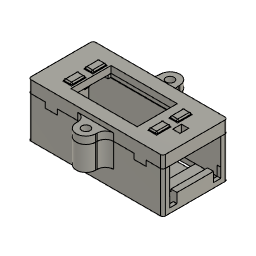
PicoCase - Display - Mounts - IO (Autodesk Fusion 360 design; units mm, degrees)
part number: PicoCase - Display - ExtraIO - Mounting Brackets - Buttons
Autodesk Fusion 360 part; units mm, degrees
note: some values were not read from the file. Set by a fixed rule: which sketch regions a step uses.
sketch "Base" plane through (0, 0, 0) normal (0, 0, 1) x (1, 0, 0)
  line L0 (1, 0) -> (54.5, 0)
  line L1 (55.5, 1) -> (55.5, 25.7)
  line L2 (54.5, 26.7) -> (1, 26.7)
  line L3 (0, 25.7) -> (0, 1)
  arc A0 (1, 26.7) -> (0, 25.7) centre (1, 25.7) ccw
  arc A1 (55.5, 25.7) -> (54.5, 26.7) centre (54.5, 25.7) ccw
  arc A2 (54.5, 0) -> (55.5, 1) centre (54.5, 1) ccw
  arc A3 (0, 1) -> (1, 0) centre (1, 1) ccw
  line L4 (1, 25.7) -> (1, 1)
  line L5 (54, 23.9) -> (55.5, 23.9)
  line L6 (53, 2.8) -> (55.5, 2.8)
  line L7 (1, 25.7) -> (53, 25.7)
  line L8 (53, 25.7) -> (53, 23.9)
  line L9 (53, 23.9) -> (1, 23.9)
  line L10 (1, 23.9) -> (1, 25.7)
  line L11 (1, 23.9) -> (54, 23.9)
  line L12 (54, 23.89) -> (1, 23.89)
  line L13 (1, 23.89) -> (1, 23.9)
  line L14 (1, 23.89) -> (54, 23.89)
  line L15 (54, 23.89) -> (54, 20.89)
  line L16 (54, 20.89) -> (1, 20.89)
  line L17 (1, 20.89) -> (1, 23.89)
  line L18 (54, 23.9) -> (54, 23.89)
  line L19 (1, 20.89) -> (53, 20.89)
  line L20 (53, 20.89) -> (53, 5.81)
  line L21 (53, 5.81) -> (1, 5.81)
  line L22 (1, 5.81) -> (1, 20.89)
  line L23 (48, 20.89) -> (53, 20.89)
  line L24 (53, 20.89) -> (53, 5.81)
  line L25 (53, 5.81) -> (48, 5.81)
  line L26 (48, 5.81) -> (48, 20.89)
  line L27 (1, 2.8) -> (53, 2.8)
  line L28 (53, 2.8) -> (53, 1)
  line L29 (53, 1) -> (1, 1)
  line L30 (1, 1) -> (1, 2.8)
  line L31 (1, 2.81) -> (54, 2.81)
  line L32 (54, 2.81) -> (54, 2.8)
  line L33 (54, 2.8) -> (1, 2.8)
  line L34 (1, 2.8) -> (1, 2.81)
  line L35 (1, 5.81) -> (54, 5.81)
  line L36 (54, 5.81) -> (54, 2.81)
  line L37 (54, 2.81) -> (1, 2.81)
  line L38 (1, 2.81) -> (1, 5.81)
  circle A4 centre (27.75, 30.7) radius 1.7
  line L39 (31.75, 30.7) -> (31.75, 26.7)
  line L40 (23.75, 30.7) -> (23.75, 26.7)
  arc A5 (31.75, 30.7) -> (23.75, 30.7) centre (27.75, 30.7) ccw
  line L41 (27.75, 30.7) -> (27.75, 26.7) construction
  circle A6 centre (27.75, -4) radius 1.7
  line L42 (27.75, -4) -> (27.75, 0) construction
  line L43 (23.75, -4) -> (23.75, 0)
  line L44 (31.75, -4) -> (31.75, 0)
  arc A7 (23.75, -4) -> (31.75, -4) centre (27.75, -4) ccw
  line L45 (0, 0) -> (75, 0) construction
  line L46 (75, 0) -> (130.5, 0)
  line L47 (130.5, 0) -> (130.5, 26.7)
  line L48 (130.5, 26.7) -> (75, 26.7)
  line L49 (75, 26.7) -> (75, 0)
  line L50 (81.9375, 26.7) -> (86.9375, 26.7)
  line L51 (86.9375, 26.7) -> (86.9375, 25.7)
  line L52 (86.9375, 25.7) -> (81.9375, 25.7)
  line L53 (81.9375, 25.7) -> (81.9375, 26.7)
  line L54 (86.9375, 1) -> (86.9375, 0)
  line L55 (81.9375, 0) -> (81.9375, 1)
  line L56 (81.9375, 1) -> (86.9375, 1)
  line L57 (86.9375, 0) -> (81.9375, 0)
  line L58 (118.5625, 26.7) -> (123.5625, 26.7)
  line L59 (123.5625, 26.7) -> (123.5625, 25.7)
  line L60 (123.5625, 25.7) -> (118.5625, 25.7)
  line L61 (118.5625, 25.7) -> (118.5625, 26.7)
  line L62 (118.5625, 1) -> (123.5625, 1)
  line L63 (123.5625, 1) -> (123.5625, 0)
  line L64 (123.5625, 0) -> (118.5625, 0)
  line L65 (118.5625, 0) -> (118.5625, 1)
  line L66 (75, 23.3625) -> (76, 23.3625)
  line L67 (76, 23.3625) -> (76, 18.3625)
  line L68 (76, 18.3625) -> (75, 18.3625)
  line L69 (75, 18.3625) -> (75, 23.3625)
  line L70 (75, 8.3375) -> (76, 8.3375)
  line L71 (76, 8.3375) -> (76, 3.3375)
  line L72 (76, 3.3375) -> (75, 3.3375)
  line L73 (75, 3.3375) -> (75, 8.3375)
  line L74 (86.7, 22.35) -> (118.2, 22.35)
  line L75 (118.2, 22.35) -> (118.2, 4.35)
  line L76 (118.2, 4.35) -> (86.7, 4.35)
  line L77 (86.7, 4.35) -> (86.7, 22.35)
  line L78 (75, 13.35) -> (130.5, 13.35) construction
  line L79 (82.7, 21.2) -> (82.7, 5.7) construction
  line L80 (82.7, 21.2) -> (86.7, 21.2)
  line L81 (86.7, 21.2) -> (86.7, 14.4)
  line L82 (86.7, 14.4) -> (82.7, 14.4)
  line L83 (82.7, 14.4) -> (82.7, 21.2)
  line L84 (82.7, 12.5) -> (86.7, 12.5)
  line L85 (86.7, 12.5) -> (86.7, 5.7)
  line L86 (86.7, 5.7) -> (82.7, 5.7)
  line L87 (82.7, 5.7) -> (82.7, 12.5)
  line L88 (118.2, 21.2) -> (122.2, 21.2)
  line L89 (122.2, 21.2) -> (122.2, 14.4)
  line L90 (122.2, 14.4) -> (118.2, 14.4)
  line L91 (118.2, 14.4) -> (118.2, 21.2)
  line L92 (118.2, 12.5) -> (122.2, 12.5)
  line L93 (122.2, 12.5) -> (122.2, 5.7)
  line L94 (122.2, 5.7) -> (118.2, 5.7)
  line L95 (118.2, 5.7) -> (118.2, 12.5)
  line L96 (123, 15.15) -> (126, 15.15)
  line L97 (126, 15.15) -> (126, 11.55)
  line L98 (126, 11.55) -> (123, 11.55)
  line L99 (123, 11.55) -> (123, 15.15)
  line L100 (102.45, 22.35) -> (102.45, 4.35) construction
  line L101 (118.2, 20.8) -> (121.8, 20.8)
  line L102 (121.8, 20.8) -> (121.8, 14.8)
  line L103 (121.8, 14.8) -> (118.2, 14.8)
  line L104 (118.2, 12.1) -> (121.8, 12.1)
  line L105 (121.8, 12.1) -> (121.8, 6.1)
  line L106 (121.8, 6.1) -> (118.2, 6.1)
  line L107 (86.7, 20.8) -> (83.1, 20.8)
  line L108 (83.1, 20.8) -> (83.1, 14.8)
  line L109 (83.1, 14.8) -> (86.7, 14.8)
  line L110 (86.7, 12.1) -> (83.1, 12.1)
  line L111 (83.1, 12.1) -> (83.1, 6.1)
  line L112 (83.1, 6.1) -> (86.7, 6.1)
  line L113 (87.5, 21.6) -> (114.8, 21.6)
  line L114 (114.8, 21.6) -> (114.8, 5.1)
  line L115 (114.8, 5.1) -> (87.5, 5.1)
  line L116 (87.5, 5.1) -> (87.5, 21.6)
  line L117 (101.15, 21.6) -> (101.15, 5.1) construction
  circle A8 centre (102.75, -4) radius 1.7
  line L118 (102.75, -4) -> (102.75, 0) construction
  line L119 (98.75, -4) -> (98.75, 0)
  line L120 (106.75, -4) -> (106.75, 0)
  arc A9 (98.75, -4) -> (106.75, -4) centre (102.75, -4) ccw
  circle A10 centre (102.75, 30.7) radius 1.7
  line L121 (102.75, 30.7) -> (102.75, 26.7) construction
  line L122 (98.75, 30.7) -> (98.75, 26.7)
  line L123 (106.75, 30.7) -> (106.75, 26.7)
  arc A11 (106.75, 30.7) -> (98.75, 30.7) centre (102.75, 30.7) ccw
  line L124 (0, 0) -> (0, -20) construction
  line L125 (0, -20) -> (0.4, -20)
  line L126 (0.4, -20) -> (0.4, -23.4)
  line L127 (0.4, -23.4) -> (0, -23.4)
  line L128 (0, -23.4) -> (0, -20)
  line L129 (0, -23.4) -> (6.6, -23.4)
  line L130 (6.2, -23.4) -> (6.6, -23.4)
  line L131 (6.6, -23.4) -> (6.6, -20)
  line L132 (6.6, -20) -> (6.2, -20)
  line L133 (6.2, -20) -> (6.2, -23.4)
  line L134 (0.4, -20) -> (6.2, -20)
  line L135 (85.7, 14.4) -> (85.7, 12.5)
  point P0 (55.5, 0)
  point P1 (55.5, 26.7)
  point P2 (0, 26.7)
  point P3 (27.75, 26.7)
  point P4 (27.75, 0)
  point P5 (123, 13.35)
  point P6 (102.45, 13.35)
  point P7 (101.15, 13.35)
  dimension "d27" = 1
  dimension "d31" = 52
  dimension "d32" = 1.8
  dimension "d33" = 0.01
  dimension "d35" = 1
  dimension "d37" = 1
  dimension "d38" = 53
  dimension "d39" = 3
  dimension "d40" = 5
  dimension "d41" = 52
  dimension "d43" = 1
  dimension "d44" = 1.8
  dimension "d45" = 0.01
  dimension "d46" = 3
  dimension "d47" = 53
  dimension "d48" = 52
  dimension "d91" = 2.5
  dimension "d93" = 24.7
  dimension "d114" = 21.1
  dimension "d115" = 26.7
  dimension "d117" = 1.5
  dimension "d118" = 55.5
  dimension "d119" = 8
  dimension "d122" = 3.4
  dimension "d123" = 4
  dimension "d124" = 4
  dimension "d125" = 3.4
  dimension "d126" = 8
  dimension "d127" = 4
  dimension "d128" = 4
  dimension "d159" = 75
  dimension "d160" = 26.7
  dimension "d161" = 55.5
  dimension "d162" = 1
  dimension "d163" = 5
  dimension "d164" = 6.9375
  dimension "d165" = 1
  dimension "d166" = 5
  dimension "d167" = 6.9375
  dimension "d168" = 5
  dimension "d169" = 1
  dimension "d170" = 6.9375
  dimension "d171" = 6.9375
  dimension "d172" = 5
  dimension "d173" = 1
  dimension "d174" = 5
  dimension "d175" = 3.3375
  dimension "d176" = 1
  dimension "d177" = 5
  dimension "d178" = 3.3375
  dimension "d179" = 1
  dimension "d183" = 18
  dimension "d187" = 7.7
  dimension "d192" = 6.8
  dimension "d193" = 4
  dimension "d200" = 6.8
  dimension "d201" = 4
  dimension "d206" = 6.8
  dimension "d207" = 4
  dimension "d208" = 4
  dimension "d209" = 6.8
  dimension "d210" = 0
  dimension "d215" = 3
  dimension "d216" = 3.6
  dimension "d225" = 5.5
  dimension "d227" = 5.5
  dimension "d230" = 5.7
  dimension "d231" = 5.7
  dimension "d237" = 48
  dimension "d241" = 0.4
  dimension "d242" = 0.4
  dimension "d243" = 0.4
  dimension "d244" = 0.4
  dimension "d245" = 0.4
  dimension "d246" = 0.4
  dimension "d247" = 0.4
  dimension "d248" = 0.4
  dimension "d249" = 0.4
  dimension "d250" = 0.4
  dimension "d251" = 0.4
  dimension "d252" = 0.4
  dimension "d265" = 16.5
  dimension "d266" = 27.3
  dimension "d300" = 3.4
  dimension "d301" = 8
  dimension "d302" = 4
  dimension "d303" = 4
  dimension "d304" = 8
  dimension "d305" = 3.4
  dimension "d306" = 4
  dimension "d307" = 4
  dimension "d314" = 3.4
  dimension "d319" = 0.4
  dimension "d321" = 0.4
  dimension "d322" = 20
  dimension "d354" = 8.3
  dimension "d356" = 12.5
  dimension "d357" = 3
  dimension "d364" = 5.8
  constraint horizontal L0
  constraint vertical L1
  constraint horizontal L2
  constraint vertical L3
  constraint coincident P2 L2
  constraint coincident P2 L3
  constraint tangent L2 A0
  constraint tangent L3 A0
  constraint coincident P1 L1
  constraint coincident P1 L2
  constraint tangent L1 A1
  constraint tangent L2 A1
  constraint equal A0 A1
  constraint coincident P0 L0
  constraint coincident P0 L1
  constraint tangent L0 A2
  constraint tangent L1 A2
  constraint equal A0 A2
  constraint tangent L0 A3
  constraint tangent L3 A3
  constraint equal A0 A3
  constraint coincident L45.start L3
  constraint coincident L45.start L0
  constraint coincident L1 L5.end
  constraint perpendicular L1 L5
  constraint coincident L1 L6.end
  constraint perpendicular L1 L6
  constraint horizontal L7
  constraint vertical L8
  constraint horizontal L9
  constraint vertical L10
  constraint collinear L4 L10
  constraint horizontal L11
  constraint horizontal L12
  constraint vertical L13
  constraint collinear L4 L13
  constraint collinear L9 L11
  constraint horizontal L14
  constraint vertical L15
  constraint horizontal L16
  constraint vertical L17
  constraint collinear L4 L17
  constraint parallel L3 L4
  constraint coincident L5 L8.end
  constraint collinear L12 L14
  constraint perpendicular L12 L18
  constraint coincident L9 L5.start
  constraint coincident L12.start L14.end
  constraint horizontal L19
  constraint vertical L20
  constraint horizontal L21
  constraint vertical L22
  constraint collinear L4 L22
  constraint horizontal L23
  constraint vertical L24
  constraint horizontal L25
  constraint vertical L26
  constraint collinear L19 L23
  constraint collinear L20 L24
  constraint collinear L21 L25
  constraint collinear L16 L19
  constraint horizontal L27
  constraint vertical L28
  constraint horizontal L29
  constraint vertical L30
  constraint collinear L4 L30
  constraint coincident L6 L27.end
  constraint coincident L6.start L27.end
  constraint horizontal L31
  constraint vertical L32
  constraint horizontal L33
  constraint vertical L34
  constraint collinear L4 L34
  constraint collinear L27 L33
  constraint horizontal L35
  constraint vertical L36
  constraint horizontal L37
  constraint vertical L38
  constraint collinear L4 L38
  constraint coincident L32 L31.end
  constraint collinear L31 L37
  constraint collinear L21 L35
  constraint coincident A3.centre L29
  constraint concentric A4 A5
  constraint tangent L2 A5
  constraint coincident L2 L39.end
  constraint tangent L39 A5
  constraint coincident L2 L40.end
  constraint tangent L40 A5
  constraint coincident A4.centre A5.centre
  constraint coincident L2 P3
  constraint perpendicular L2 L41
  constraint midpoint L2 P3
  constraint coincident L41 P3
  constraint concentric A6 A7
  constraint coincident A6.centre L42.start
  constraint coincident L0 P4
  constraint perpendicular L0 L42
  constraint midpoint L0 P4
  constraint coincident L42 P4
  constraint tangent L0 A7
  constraint coincident L0 L43.end
  constraint tangent L43 A7
  constraint coincident L0 L44.end
  constraint tangent L44 A7
  constraint coincident L45.start L124.start
  constraint parallel L0 L45
  constraint horizontal L46
  constraint vertical L47
  constraint horizontal L48
  constraint vertical L49
  constraint horizontal L50
  constraint vertical L51
  constraint horizontal L52
  constraint vertical L53
  constraint collinear L48 L50
  constraint horizontal L56
  constraint vertical L54
  constraint horizontal L57
  constraint vertical L55
  constraint collinear L46 L57
  constraint horizontal L58
  constraint vertical L59
  constraint horizontal L60
  constraint vertical L61
  constraint horizontal L62
  constraint vertical L63
  constraint horizontal L64
  constraint vertical L65
  constraint collinear L48 L58
  constraint collinear L46 L64
  constraint horizontal L66
  constraint vertical L67
  constraint horizontal L68
  constraint vertical L69
  constraint horizontal L70
  constraint vertical L71
  constraint horizontal L72
  constraint vertical L73
  constraint collinear L49 L69
  constraint collinear L49 L73
  constraint horizontal L74
  constraint vertical L75
  constraint horizontal L76
  constraint vertical L77
  constraint midpoint L49 L78.start
  constraint midpoint L47 L78.end
  constraint perpendicular L78 L79
  constraint horizontal L80
  constraint vertical L81
  constraint horizontal L82
  constraint vertical L83
  constraint coincident L79.start L80
  constraint collinear L79 L83
  constraint horizontal L84
  constraint vertical L85
  constraint horizontal L86
  constraint vertical L87
  constraint coincident L79.end L86
  constraint collinear L79 L87
  constraint horizontal L88
  constraint vertical L89
  constraint horizontal L90
  constraint vertical L91
  constraint horizontal L92
  constraint vertical L93
  constraint horizontal L94
  constraint vertical L95
  constraint collinear L91 L95
  constraint horizontal L96
  constraint vertical L97
  constraint horizontal L98
  constraint vertical L99
  constraint midpoint L99 P5
  constraint coincident L78 P5
  constraint midpoint L74 L100.start
  constraint midpoint L76 L100.end
  constraint midpoint L100 P6
  constraint coincident L78 P6
  constraint horizontal L101
  constraint perpendicular L101 L102
  constraint perpendicular L102 L103
  constraint coincident L91 L101.start
  constraint coincident L91 L103.end
  constraint coincident L95 L104.start
  constraint perpendicular L95 L104
  constraint perpendicular L104 L105
  constraint coincident L95 L106.end
  constraint perpendicular L95 L106
  constraint coincident L81 L107.start
  constraint perpendicular L81 L107
  constraint perpendicular L107 L108
  constraint coincident L81 L109.end
  constraint perpendicular L81 L109
  constraint coincident L85 L110.start
  constraint perpendicular L85 L110
  constraint perpendicular L110 L111
  constraint coincident L85 L112.end
  constraint perpendicular L85 L112
  constraint collinear L77 L81
  constraint collinear L75 L91
  constraint horizontal L113
  constraint vertical L114
  constraint horizontal L115
  constraint vertical L116
  constraint midpoint L113 L117.start
  constraint midpoint L115 L117.end
  constraint midpoint L117 P7
  constraint coincident L78 P7
  constraint concentric A8 A9
  constraint coincident A8.centre L118.start
  constraint midpoint L46 L118.end
  constraint perpendicular L46 L118
  constraint coincident L46 L119.end
  constraint tangent L119 A9
  constraint coincident L46 L120.end
  constraint tangent L120 A9
  constraint perpendicular L46 L119
  constraint concentric A10 A11
  constraint coincident A10.centre L121.start
  constraint midpoint L48 L121.end
  constraint perpendicular L48 L121
  constraint coincident L48 L122.end
  constraint perpendicular L48 L122
  constraint coincident L48 L123.end
  constraint tangent L123 A11
  constraint perpendicular L48 L123
  constraint perpendicular L45 L124
  constraint horizontal L125
  constraint vertical L126
  constraint horizontal L127
  constraint vertical L128
  constraint horizontal L129
  constraint horizontal L130
  constraint vertical L131
  constraint horizontal L132
  constraint vertical L133
  constraint coincident L127.end L128.start
  constraint coincident L129.end L130.end
  constraint coincident L124.end L125.start
  constraint parallel L129 L134
  constraint coincident L82 L135.start
  constraint coincident L84 L135.end
  constraint perpendicular L84 L135
  measures "d27" radius of A0
  measures "d31" distance of L8 L10
  measures "d32" distance of L7 L9
  measures "d33" distance of L11 L12
  measures "d35" distance of L3 L4
  measures "d37" distance of L2 L7
  measures "d38" distance of L15.end L16.end
  measures "d39" distance of L14 L16
  measures "d40" distance of L24 L26
  measures "d41" distance of L28 L30
  measures "d43" distance of L0 L29
  measures "d44" distance of L27 L29
  measures "d45" distance of L31 L33
  measures "d46" distance of L35 L37
  measures "d47" distance of L36 L38
  measures "d48" distance of L22 L24
  measures "d91" distance of L1 L20
  measures "d93" distance of L7 L29
  measures "d114" distance of L9 L27
  measures "d115" distance of L0 L2
  measures "d117" distance of L1 L15
  measures "d118" distance of L1 L3
  measures "d119" diameter of A5
  measures "d122" diameter of A4
  measures "d123" vertical distance of L39.start L39.end
  measures "d124" vertical distance of L40.start L40.end
  measures "d125" diameter of A6
  measures "d126" diameter of A7
  measures "d127" vertical distance of L43.start L43.end
  measures "d128" vertical distance of L44.start L44.end
  measures "d159" distance of L45.start L45.end
  measures "d160" distance of L45.end L48.end
  measures "d161" distance of L47.end L48.end
  measures "d162" distance of L50.end L51.end
  measures "d163" distance of L51 L53
  measures "d164" distance of L49 L53
  measures "d165" distance of L54.end L54.start
  measures "d166" distance of L54 L55
  measures "d167" distance of L49 L55
  measures "d168" distance of L59 L61
  measures "d169" distance of L58 L60
  measures "d170" distance of L47 L59
  measures "d171" distance of L47 L63
  measures "d172" distance of L63 L65
  measures "d173" distance of L62 L64
  measures "d174" distance of L66 L68
  measures "d175" distance of L48 L66
  measures "d176" distance of L67 L69
  measures "d177" distance of L70 L72
  measures "d178" distance of L46 L72
  measures "d179" distance of L71 L73
  measures "d183" distance of L74 L76
  measures "d187" distance of L49 L79
  measures "d192" distance of L80 L82
  measures "d193" distance of L81 L83
  measures "d200" distance of L84 L86
  measures "d201" distance of L85 L87
  measures "d206" distance of L88 L90
  measures "d207" distance of L89 L91
  measures "d208" distance of L93 L95
  measures "d209" distance of L92 L94
  measures "d210" distance of L75 L91
  measures "d215" distance of L97 L99
  measures "d216" distance of L96 L98
  measures "d225" distance of L48 L88
  measures "d227" distance of L48 L80
  measures "d230" distance of L46 L94
  measures "d231" distance of L46 L86
  measures "d237" distance of L49 L99
  measures "d241" distance of L88 L101
  measures "d242" distance of L89 L102
  measures "d243" distance of L90 L103
  measures "d244" distance of L92 L104
  measures "d245" distance of L93 L105
  measures "d246" distance of L94 L106
  measures "d247" distance of L80 L107
  measures "d248" distance of L79 L108
  measures "d249" distance of L82 L109
  measures "d250" distance of L84 L110
  measures "d251" distance of L79 L111
  measures "d252" distance of L86 L112
  measures "d265" distance of L113 L115
  measures "d266" distance of L114 L116
  measures "d300" diameter of A8
  measures "d301" diameter of A9
  measures "d302" vertical distance of L119.start L119.end
  measures "d303" vertical distance of L120.start L120.end
  measures "d304" diameter of A11
  measures "d305" diameter of A10
  measures "d306" distance of L123.start L123.end
  measures "d307" distance of L122.start L122.end
  measures "d314" distance of L125.end L126.end
  measures "d319" distance of L126 L128
  measures "d321" distance of L131 L133
  measures "d322" distance of L45.start L124.end
  measures "d354" distance of L47 L89
  measures "d356" distance of L49 L116
  measures "d357" distance of L79 L135
  measures "d364" distance of L126 L133
extrude "Extrude1" add sketch "Base" along normal blind 17 contours L0 L1 L2 L3 A0 A1 A2 A3 L4 L5 L6 L7 L8 L10 L11 L13 L17 L22 L28 L29 L30 L33 L34 L38 makes body 1
extrude "Extrude2" add sketch "Base" along normal blind 15.25 contours L4 L7 L8 L9 L10 L11 bodies 1
extrude "Extrude3" add sketch "Base" along normal blind 2 contours L4 L9 L11 L12 L13 L14 L18 bodies 1
extrude "Extrude4" add sketch "Base" along normal blind 2 contours L4 L16 L19 L21 L22 L26 L35 bodies 1
extrude "Extrude5" add sketch "Base" along normal blind 5 contours L16 L19 L20 L21 L23 L24 L25 L26 L35 bodies 1
extrude "Extrude6" add sketch "Base" along normal blind 2 contours L4 L6 L27 L31 L32 L33 L34 L37 bodies 1
extrude "Extrude7" add sketch "Base" along normal blind 15.25 contours L4 L27 L28 L29 L30 L33 bodies 1
extrude "Extrude8" add sketch "Base" along normal blind 6 contours L1 L5 L6 L15 L16 L18 L20 L24 L32 L35 L36 bodies 1
sketch "Insert End" plane through (55.5, 0, 0) normal (1, 0, 0) x (0, 1, 0)
  line L0 (1, 0) -> (25.7, 0)
  line L1 (25.7, 0) -> (25.7, 17)
  line L2 (25.7, 17) -> (23.9, 17)
  line L3 (23.9, 17) -> (23.9, 6)
  line L4 (23.9, 6) -> (2.8, 6)
  line L5 (2.8, 6) -> (2.8, 17)
  line L6 (2.8, 17) -> (1, 17)
  line L7 (1, 17) -> (1, 0)
  line L8 (2.81, 6) -> (5.81, 6)
  line L9 (5.81, 6) -> (5.81, 2)
  line L10 (5.81, 2) -> (2.81, 2)
  line L11 (2.81, 2) -> (2.81, 6)
  line L12 (1, 0) -> (25.7, 0)
  line L13 (20.89, 6) -> (23.89, 6)
  line L14 (23.89, 6) -> (23.89, 2)
  line L15 (23.89, 2) -> (20.89, 2)
  line L16 (20.89, 2) -> (20.89, 6)
  point P0 (26.7, 0)
  dimension "d66" = 3
  dimension "d67" = 2.81
  dimension "d68" = 2
  dimension "d69" = 2
  dimension "d70" = 3
  dimension "d71" = 2.81
  constraint horizontal L8
  constraint vertical L9
  constraint horizontal L10
  constraint vertical L11
  constraint collinear L4 L8
  constraint horizontal L13
  constraint vertical L14
  constraint horizontal L15
  constraint vertical L16
  constraint collinear L4 L13
  measures "d66" distance of L9 L11
  measures "d67" distance of origin L11
  measures "d68" distance of L10 L12
  measures "d69" distance of L12 L15
  measures "d70" distance of L14 L16
  measures "d71" distance of L14 P0
extrude "Extrude9" cut sketch "Insert End" against normal up to surface (1.5 mm away) contours L4 L8 L9 L10 L11 bodies 1
extrude "Extrude10" cut sketch "Insert End" against normal up to surface (1.5 mm away) contours L4 L13 L14 L15 L16 bodies 1
sketch "USB End" plane through (0, 0, 0) normal (-1, 0, 0) x (0, -1, 0)
  line L0 (-25.7, 0) -> (-1, 0)
  line L1 (-1, 0) -> (-1, 17)
  line L2 (-1, 17) -> (-25.7, 17)
  line L3 (-25.7, 17) -> (-25.7, 0)
  line L4 (-13.35, 17) -> (-13.35, 0) construction
  line L5 (-17.45, 7) -> (-9.25, 7)
  line L6 (-9.25, 7) -> (-9.25, 2)
  line L7 (-9.25, 2) -> (-17.45, 2)
  line L8 (-17.45, 2) -> (-17.45, 7)
  line L9 (-25.7, 0) -> (-1, 0)
  line L10 (-23.3625, 17) -> (-18.3625, 17)
  line L11 (-18.3625, 17) -> (-18.3625, 14.75)
  line L12 (-18.3625, 14.75) -> (-23.3625, 14.75)
  line L13 (-23.3625, 14.75) -> (-23.3625, 17)
  line L14 (-8.3375, 17) -> (-3.3375, 17)
  line L15 (-3.3375, 17) -> (-3.3375, 14.75)
  line L16 (-3.3375, 14.75) -> (-8.3375, 14.75)
  line L17 (-8.3375, 14.75) -> (-8.3375, 17)
  point P0 (-13.35, 7)
  point P1 (-26.7, 0)
  dimension "d76" = 5
  dimension "d77" = 8.2
  dimension "d78" = 2
  dimension "d79" = 2.25
  dimension "d80" = 5
  dimension "d81" = 3.3375
  dimension "d82" = 5
  dimension "d83" = 2.25
  dimension "d84" = 3.3375
  constraint midpoint L2 L4.start
  constraint midpoint L0 L4.end
  constraint horizontal L5
  constraint vertical L6
  constraint horizontal L7
  constraint vertical L8
  constraint midpoint L5 P0
  constraint coincident L4 P0
  constraint horizontal L10
  constraint vertical L11
  constraint horizontal L12
  constraint vertical L13
  constraint collinear L2 L10
  constraint horizontal L14
  constraint vertical L15
  constraint horizontal L16
  constraint vertical L17
  constraint collinear L2 L14
  measures "d76" distance of L5 L7
  measures "d77" distance of L6 L8
  measures "d78" distance of L7 L9
  measures "d79" distance of L10 L12
  measures "d80" distance of L11 L13
  measures "d81" distance of L13 P1
  measures "d82" distance of L15 L17
  measures "d83" distance of L14 L16
  measures "d84" distance of L15 origin
extrude "Extrude11" cut sketch "USB End" against normal up to surface (1 mm away) contours L5 L6 L7 L8 bodies 1
extrude "Extrude12" cut sketch "USB End" against normal up to surface (1 mm away) contours L2 L10 L11 L12 L13 bodies 1
extrude "Extrude13" cut sketch "USB End" against normal up to surface (1 mm away) contours L2 L14 L15 L16 L17 bodies 1
sketch "Front" plane through (0, 0, 0) normal (0, -1, 0) x (1, 0, 0)
  line L0 (1, 0) -> (54.5, 0)
  line L1 (54.5, 0) -> (54.5, 17)
  line L2 (54.5, 17) -> (1, 17)
  line L3 (1, 17) -> (1, 0)
  line L4 (6.9375, 17) -> (11.9375, 17)
  line L5 (11.9375, 17) -> (11.9375, 14.75)
  line L6 (11.9375, 14.75) -> (6.9375, 14.75)
  line L7 (6.9375, 14.75) -> (6.9375, 17)
  line L8 (43.5625, 17) -> (48.5625, 17)
  line L9 (48.5625, 17) -> (48.5625, 14.75)
  line L10 (48.5625, 14.75) -> (43.5625, 14.75)
  line L11 (43.5625, 14.75) -> (43.5625, 17)
  point P0 (55.5, 0)
  dimension "d94" = 2.25
  dimension "d95" = 5
  dimension "d96" = 6.9375
  dimension "d97" = 2.25
  dimension "d98" = 5
  dimension "d99" = 6.9375
  constraint horizontal L4
  constraint vertical L5
  constraint horizontal L6
  constraint vertical L7
  constraint collinear L2 L4
  constraint horizontal L8
  constraint vertical L9
  constraint horizontal L10
  constraint vertical L11
  constraint collinear L2 L8
  measures "d94" distance of L4 L6
  measures "d95" distance of L5 L7
  measures "d96" distance of L7 origin
  measures "d97" distance of L8 L10
  measures "d98" distance of L9 L11
  measures "d99" distance of L9 P0
extrude "Extrude14" cut sketch "Front" against normal up to surface (1 mm away) contours L2 L4 L5 L6 L7 bodies 1
extrude "Extrude15" cut sketch "Front" against normal up to surface (1 mm away) contours L2 L8 L9 L10 L11 bodies 1
sketch "Back" plane through (0, 26.7, 0) normal (0, 1, 0) x (-1, 0, 0)
  line L0 (-54.5, 0) -> (-1, 0)
  line L1 (-1, 0) -> (-1, 17)
  line L2 (-1, 17) -> (-54.5, 17)
  line L3 (-54.5, 17) -> (-54.5, 0)
  line L4 (-48.5625, 17) -> (-43.5625, 17)
  line L5 (-43.5625, 17) -> (-43.5625, 14.75)
  line L6 (-43.5625, 14.75) -> (-48.5625, 14.75)
  line L7 (-48.5625, 14.75) -> (-48.5625, 17)
  line L8 (-11.9375, 17) -> (-6.9375, 17)
  line L9 (-6.9375, 17) -> (-6.9375, 14.75)
  line L10 (-6.9375, 14.75) -> (-11.9375, 14.75)
  line L11 (-11.9375, 14.75) -> (-11.9375, 17)
  point P0 (-55.5, 0)
  dimension "d104" = 2.25
  dimension "d105" = 5
  dimension "d106" = 6.9375
  dimension "d107" = 5
  dimension "d108" = 2.25
  dimension "d109" = 6.9375
  constraint horizontal L4
  constraint vertical L5
  constraint horizontal L6
  constraint vertical L7
  constraint collinear L2 L4
  constraint horizontal L8
  constraint vertical L9
  constraint horizontal L10
  constraint vertical L11
  constraint collinear L2 L8
  measures "d104" distance of L4 L6
  measures "d105" distance of L5 L7
  measures "d106" distance of L7 P0
  measures "d107" distance of L9 L11
  measures "d108" distance of L8 L10
  measures "d109" distance of origin L9
extrude "Extrude16" cut sketch "Back" against normal up to surface (1 mm away) contours L2 L8 L9 L10 L11 bodies 1
extrude "Extrude17" cut sketch "Back" against normal up to surface (1 mm away) contours L2 L4 L5 L6 L7 bodies 1
extrude "Extrude18" add sketch "Base" along normal up to surface (10 mm away) from surface at 7 contours L0 L43 L44 A7 bodies 1
fillet "Fillet1" radius 3.4 1 edges at (23.75, 0, 12) on bodies 1
fillet "Fillet2" radius 3.4 1 edges at (31.75, 0, 12) on bodies 1
extrude "Extrude19" add sketch "Base" along normal up to surface (10 mm away) from surface at 7 contours L2 L39 L40 A5 bodies 1
fillet "Fillet3" radius 3.4 1 edges at (31.75, 26.7, 12) on bodies 1
fillet "Fillet4" radius 3.4 1 edges at (23.75, 26.7, 12) on bodies 1
sketch "Underside Mount" plane through (0, 0, 7) normal (0, 0, -1) x (1, 0, 0)
  circle A0 centre (27.75, -30.7) radius 1.7
  line L0 (35.15, -26.7) -> (20.35, -26.7)
  arc A1 (23.75, -30.1) -> (20.35, -26.7) centre (20.35, -30.1) ccw
  arc A2 (23.75, -30.7) -> (31.75, -30.7) centre (27.75, -30.7) ccw
  arc A3 (35.15, -26.7) -> (31.75, -30.1) centre (35.15, -30.1) ccw
  line L1 (31.2141, -30.7) -> (29.4821, -27.7)
  line L2 (29.4821, -27.7) -> (26.0179, -27.7)
  line L3 (26.0179, -27.7) -> (24.2859, -30.7)
  line L4 (24.2859, -30.7) -> (26.0179, -33.7)
  line L5 (26.0179, -33.7) -> (29.4821, -33.7)
  line L6 (29.4821, -33.7) -> (31.2141, -30.7)
  line L7 (54.5, -26.7) -> (1, -26.7)
  line L8 (29.4821, 1) -> (31.2141, 4)
  line L9 (31.2141, 4) -> (29.4821, 7)
  line L10 (29.4821, 7) -> (26.0179, 7)
  line L11 (26.0179, 7) -> (24.2859, 4)
  line L12 (24.2859, 4) -> (26.0179, 1)
  line L13 (26.0179, 1) -> (29.4821, 1)
  line L14 (1, 0) -> (54.5, 0)
  line L15 (31.75, -30.7) -> (31.75, -30.1)
  line L16 (23.75, -30.1) -> (23.75, -30.7)
  point P0 (27.75, -30.7)
  point P1 (27.75, -30.7)
  point P2 (27.75, 4)
  point P3 (27.75, 4)
  dimension "d157" = 6
  dimension "d158" = 6
  constraint parallel L2 L7
  constraint coincident P1 P0
  constraint parallel L13 L14
  constraint coincident P3 P2
  measures "d157" distance of L10 L13
  measures "d158" distance of L2 L5
extrude "Extrude20" cut sketch "Underside Mount" against normal blind 2.4 contours L8 L9 L10 L11 L12 L13 bodies 1
extrude "Extrude21" cut sketch "Underside Mount" against normal blind 2.4 contours L1 L2 L3 L4 L5 L6 bodies 1
extrude "Extrude22" add sketch "Base" along normal blind 5 separate body contours L46 L47 L48 L49 L51 L52 L53 L54 L55 L56 L59 L60 L61 L62 L63 L65 L66 L67 L68 L70 L71 L72 | L77 L82 L84 L135 makes body 2
extrude "Extrude23" add sketch "Base" along normal blind 5 contours L46 L54 L55 L56 L57 bodies 2
extrude "Extrude24" add sketch "Base" against normal blind 2.25 contours L46 L54 L55 L56 L57 bodies 2
extrude "Extrude25" add sketch "Base" along normal up to surface (2.2 mm away) from surface at 2.8 contours L77 L84 L85 L86 L87 L110 L111 L112 bodies 2
extrude "Extrude26" add sketch "Base" along normal up to surface (2.8 mm away) from surface at 2.2 separate body contours L74 L75 L76 L77 L81 L85 L91 L95 makes body 3
extrude "Extrude27" add sketch "Base" along normal up to surface (2.2 mm away) from surface at 2.8 contours L77 L80 L81 L82 L83 L107 L108 L109 bodies 2 3
extrude "Extrude28" add sketch "Base" along normal up to surface (2.2 mm away) from surface at 2.8 contours L75 L88 L89 L90 L91 L101 L102 L103 bodies 2
extrude "Extrude29" add sketch "Base" along normal up to surface (2.2 mm away) from surface at 2.8 contours L75 L92 L93 L94 L95 L104 L105 L106 bodies 2
extrude "Extrude30" add sketch "Base" along normal up to surface (5 mm away) contours L49 L70 L71 L72 L73 bodies 2
extrude "Extrude31" add sketch "Base" along normal up to surface (5 mm away) contours L49 L66 L67 L68 L69 bodies 2
extrude "Extrude32" add sketch "Base" along normal up to surface (5 mm away) contours L48 L50 L51 L52 L53 bodies 2
extrude "Extrude33" add sketch "Base" along normal up to surface (5 mm away) contours L48 L58 L59 L60 L61 bodies 2
extrude "Extrude34" add sketch "Base" along normal up to surface (5 mm away) contours L46 L62 L63 L64 L65 bodies 2
extrude "Extrude35" add sketch "Base" against normal blind 2.25 contours L46 L62 L63 L64 L65 bodies 2
extrude "Extrude36" add sketch "Base" against normal blind 2.25 contours L48 L58 L59 L60 L61 bodies 2
extrude "Extrude37" add sketch "Base" against normal blind 2.25 contours L48 L50 L51 L52 L53 bodies 2
extrude "Extrude38" add sketch "Base" against normal blind 2.25 contours L49 L66 L67 L68 L69 bodies 2
extrude "Extrude39" add sketch "Base" against normal blind 2.25 contours L49 L70 L71 L72 L73 bodies 2
extrude "Extrude40" add sketch "Base" along normal blind 3 contours L46 L119 L120 A9 bodies 2
extrude "Extrude41" add sketch "Base" along normal blind 3 contours L48 L122 L123 A11 bodies 2
extrude "Extrude42" add sketch "Base" along normal blind 1 separate body contours L125 L126 L127 L128 L129 makes body 4
extrude "Extrude44" add sketch "Base" along normal blind 1 separate body contours L129 L130 L131 L132 L133 makes body 5
extrude "Extrude45" add sketch "Base" along normal blind 2 from surface at 2 separate body contours L126 L129 L133 L134 makes body 6
fillet "Fillet5" radius 0.5 8 edges at (6.2, -21.7, 4) (3.3, -23.4, 4) (0.4, -21.7, 4) (3.3, -20, 4) (6.2, -23.4, 3) (0.4, -23.4, 3) (0.4, -20, 3) (6.2, -20, 3) on bodies 6
extrude "Extrude46" add sketch "Base" along normal blind 1.5 from surface at 0.7 contours L126 L129 L133 L134 bodies 6 4 5
fillet "Fillet7" radius 3.4 1 edges at (106.75, 0, 1.5) on bodies 2
fillet "Fillet8" radius 3.4 1 edges at (98.75, 0, 1.5) on bodies 2
fillet "Fillet9" radius 3.4 1 edges at (98.75, 26.7, 1.5) on bodies 2
fillet "Fillet10" radius 3.4 1 edges at (106.75, 26.7, 1.5) on bodies 2
extrude "Extrude48" cut sketch "Base" along normal blind 2.2 contours L77 L82 L84 L135 bodies 2
copy_body "Body->Comp1" bodies 2 removing the originals makes body 7 in component "Top"
copy_body "Body->Comp2" bodies 1 removing the originals makes body 8 in component "Base"
copy_body "Body->Comp3" bodies 6 removing the originals makes body 9 in component "Button"
move_body "Move1" bodies 7 to x (1, 0, 0) y (0, 1, 0) z (0, 0, 1) at (5, -25, 30) in component "Top"
sketch "Sketch1" plane through (0, 0, 0) normal (0, 0, 1) x (1, 0, 0) in component "PCB Button"
  line L0 (41.7, -17.9) -> (45, -17.9)
  line L1 (45, -17.9) -> (45, -22.1)
  line L2 (45, -22.1) -> (41.7, -22.1)
  line L3 (41.7, -22.1) -> (41.7, -17.9)
  line L4 (42.75, -18.5) -> (43.95, -18.5)
  line L5 (44.45, -19) -> (44.45, -21)
  line L6 (43.95, -21.5) -> (42.75, -21.5)
  line L7 (42.25, -21) -> (42.25, -19)
  arc A0 (44.45, -19) -> (43.95, -18.5) centre (43.95, -19) ccw
  arc A1 (43.95, -21.5) -> (44.45, -21) centre (43.95, -21) ccw
  arc A2 (42.25, -21) -> (42.75, -21.5) centre (42.75, -21) ccw
  arc A3 (42.75, -18.5) -> (42.25, -19) centre (42.75, -19) ccw
  line L8 (43.35, -18.5) -> (43.35, -21.5) construction
  line L9 (42.25, -20) -> (44.45, -20) construction
  line L10 (41.7, -20) -> (45, -20) construction
  line L11 (43.35, -17.9) -> (43.35, -22.1) construction
  point P0 (43.35, -20)
  dimension "d365" = 4.2
  dimension "d366" = 3.3
  dimension "d367" = 3
  dimension "d368" = 2.2
  dimension "d369" = 0.5
  constraint horizontal L0
  constraint vertical L1
  constraint horizontal L2
  constraint vertical L3
  constraint horizontal L4
  constraint vertical L5
  constraint horizontal L6
  constraint vertical L7
  constraint tangent L4 A0
  constraint tangent L5 A0
  constraint tangent L5 A1
  constraint tangent L6 A1
  constraint equal A0 A1
  constraint tangent L6 A2
  constraint tangent L7 A2
  constraint equal A0 A2
  constraint tangent L4 A3
  constraint tangent L7 A3
  constraint equal A0 A3
  constraint midpoint L4 L8.start
  constraint midpoint L6 L8.end
  constraint midpoint L7 L9.start
  constraint midpoint L5 L9.end
  constraint midpoint L3 L10.start
  constraint midpoint L1 L10.end
  constraint midpoint L0 L11.start
  constraint midpoint L2 L11.end
  constraint midpoint L8 P0
  constraint coincident L10 P0
  constraint coincident L11 P0
  measures "d365" distance of L0 L2
  measures "d366" distance of L1 L3
  measures "d367" distance of L4 L6
  measures "d368" distance of L5 L7
  measures "d369" radius of A0
extrude "Extrude1'" add sketch "Sketch1" along normal blind 1.85 separate body makes body 10 in component "PCB Button"
extrude "Extrude2'" add sketch "Sketch1" along normal blind 2.5 contours L4 L5 L6 L7 A0 A1 A2 A3 bodies 10 in component "PCB Button"
ref_plane "WorkPlane1" through (107.75, -11.65, 30) normal (0, 0, -1) x (-1, 0, 0) in component "Top"
sketch "Button Hole Projection" plane through (107.75, -11.65, 30) normal (0, 0, -1) x (1, 0, 0) in component "Top"
  line L0 (-16.05, -7.45) -> (-19.65, -7.45)
  line L1 (-19.65, -7.45) -> (-19.65, -1.45)
  line L2 (-16.05, -1.45) -> (-16.05, -7.45)
  line L3 (-19.65, -1.45) -> (-16.05, -1.45)
  line L4 (-16.05, 1.25) -> (-19.65, 1.25)
  line L5 (-19.65, 7.25) -> (-16.05, 7.25)
  line L6 (-19.65, 1.25) -> (-19.65, 7.25)
  line L7 (-16.05, 7.25) -> (-16.05, 1.25)
  line L8 (19.05, -7.45) -> (15.45, -7.45)
  line L9 (15.45, -1.45) -> (19.05, -1.45)
  line L10 (15.45, -7.45) -> (15.45, -1.45)
  line L11 (19.05, -1.45) -> (19.05, -7.45)
  line L12 (19.05, 1.25) -> (15.45, 1.25)
  line L13 (19.05, 7.25) -> (19.05, 1.25)
  line L14 (15.45, 1.25) -> (15.45, 7.25)
  line L15 (15.45, 7.25) -> (19.05, 7.25)
fillet "Fillet1'" radius 1 1 edges at (80, -25, 32.5) on bodies 7 in component "Top"
fillet "Fillet2'" radius 1 1 edges at (80, 1.7, 32.5) on bodies 7 in component "Top"
fillet "Fillet3'" radius 1 1 edges at (135.5, -25, 32.5) on bodies 7 in component "Top"
fillet "Fillet4'" radius 1 1 edges at (135.5, 1.7, 32.5) on bodies 7 in component "Top"
component "Base" placed x (1, 0, 0) y (0, 1, 0) z (0, 0, 1) at (0, 0, 0)
component "Top" placed x (1, 0, 0) y (0, 1, 0) z (0, 0, 1) at (-80, 25, -13)
component "Button" placed x (0, 1, 0) y (-1, 0, 0) z (0, 0, 1) at (23.3, 14.5, 18.8)
component "PCB Button" placed x (1, 0, 0) y (0, 1, 0) z (0, 0, 1) at (1.5, 29.1, 17)
component "Button" placed x (0, 1, 0) y (-1, 0, 0) z (0, 0, 1) at (23.3, 5.8, 18.8)
component "PCB Button" placed x (1, 0, 0) y (0, 1, 0) z (0, 0, 1) at (1.5, 37.8, 17)
component "PCB Button" placed x (1, 0, 0) y (0, 1, 0) z (0, 0, 1) at (-33.3, 29.1, 17)
component "PCB Button" placed x (1, 0, 0) y (0, 1, 0) z (0, 0, 1) at (-33.3, 37.8, 17)
component "Button" placed x (0, 1, 0) y (-1, 0, 0) z (0, 0, 1) at (-11.8, 14.5, 18.8)
component "Button" placed x (0, 1, 0) y (-1, 0, 0) z (0, 0, 1) at (-11.8, 5.8, 18.8)
equation "boardsHeight = 12 mm + usbHeight"
equation "usbHeight = 3 mm"
equation "boardWidth = 21.1 mm"
equation "boardLength = 52 mm"
equation "insetWidth = 1.8 mm"
equation "wallThickness = 1 mm"
equation "cornerRadius = 1 mm"
equation "ioGap = 3 mm"
equation "usbHoleHeight = 5 mm"
equation "usbHoleWdith = 8.2 mm"
equation "baseThickness = 2 mm"
equation "endHeight = 4 mm + baseThickness"
equation "ioLength = 53 mm"
equation "insetDepth = 1.75 mm"
equation "tabWidth = 5 mm"
equation "tabHeight = insetDepth + 0.5 mm"
equation "insetHeight = baseThickness + boardsHeight - insetDepth"
equation "displayLength = 52 mm"
equation "supportHeight = baseThickness + usbHeight"
equation "supportWidth = 5 mm"
equation "length = ioLength + wallThickness + 1.5 mm"
equation "height = boardsHeight + baseThickness"
equation "width = boardWidth + 2 * ( wallThickness + insetWidth )"
equation "ioOffset = 0.01 mm"
equation "d27 = cornerRadius"
equation "d31 = displayLength"
equation "d32 = insetWidth"
equation "d33 = ioOffset"
equation "d35 = wallThickness"
equation "d37 = wallThickness"
equation "d38 = ioLength"
equation "d39 = ioGap"
equation "d40 = supportWidth"
equation "d41 = displayLength"
equation "d43 = wallThickness"
equation "d44 = insetWidth"
equation "d45 = ioOffset"
equation "d46 = ioGap"
equation "d47 = ioLength"
equation "d48 = boardLength"
equation "d49 = height"
equation "d51 = insetHeight"
equation "d53 = baseThickness"
equation "d55 = baseThickness"
equation "d57 = supportHeight"
equation "d59 = baseThickness"
equation "d61 = insetHeight"
equation "d63 = endHeight"
equation "d66 = ioGap"
equation "d67 = wallThickness + insetWidth + ioOffset"
equation "d68 = baseThickness"
equation "d69 = baseThickness"
equation "d70 = ioGap"
equation "d71 = wallThickness + insetWidth + ioOffset"
equation "d76 = usbHoleHeight"
equation "d77 = usbHoleWdith"
equation "d78 = baseThickness"
equation "d79 = tabHeight"
equation "d80 = tabWidth"
equation "d81 = width / 8"
equation "d82 = tabWidth"
equation "d83 = tabHeight"
equation "d84 = width / 8"
equation "d94 = tabHeight"
equation "d95 = tabWidth"
equation "d96 = length / 8"
equation "d97 = tabHeight"
equation "d98 = tabWidth"
equation "d99 = length / 8"
equation "d104 = tabHeight"
equation "d105 = tabWidth"
equation "d106 = length / 8"
equation "d107 = tabWidth"
equation "d108 = tabHeight"
equation "d109 = length / 8"
equation "d114 = boardWidth"
equation "endJoinWidth = 1.5 mm"
equation "d117 = endJoinWidth"
equation "d119 = mountOD"
equation "mountOD = nutWidth + 2 mm"
equation "mountID = 3.4 mm"
equation "d122 = mountID"
equation "d123 = mountOD / 2"
equation "d124 = mountOD / 2"
equation "d125 = mountID"
equation "d126 = mountOD"
equation "d127 = mountOD / 2"
equation "d128 = mountOD / 2"
equation "d131 = height - baseMountLength"
equation "baseMountLength = 10 mm"
equation "d134 = mountID"
equation "d136 = mountID"
equation "d137 = height - baseMountLength"
equation "d141 = mountID"
equation "d143 = mountID"
equation "nutWidth = 6 mm"
equation "nutHeight = 2.4 mm"
equation "d149 = -nutHeight"
equation "d151 = -nutHeight"
equation "d157 = nutWidth"
equation "d158 = nutWidth"
equation "d160 = width"
equation "d161 = length"
equation "d162 = wallThickness"
equation "d163 = tabWidth"
equation "d164 = length / 8"
equation "d165 = wallThickness"
equation "d166 = tabWidth"
equation "d167 = length / 8"
equation "d168 = tabWidth"
equation "d169 = wallThickness"
equation "d170 = length / 8"
equation "d171 = length / 8"
equation "d172 = tabWidth"
equation "d173 = wallThickness"
equation "d174 = tabWidth"
equation "d175 = width / 8"
equation "d176 = wallThickness"
equation "d177 = tabWidth"
equation "d178 = width / 8"
equation "d179 = wallThickness"
equation "topThickness = 5 mm"
equation "d183 = screenHeight"
equation "screenLeftOffset = 11.5 mm + wallThickness"
equation "screenHeight = 18 mm"
equation "visibleScreenWidth = 27.3 mm"
equation "d187 = buttonLeftOffset"
equation "buttonLeftOffset = 7.7 mm"
equation "buttonHoleWidth = 4 mm"
equation "buttonHoleLength = 6.8 mm"
equation "d192 = buttonHoleLength"
equation "d193 = buttonHoleWidth"
equation "buttonHorizontaSpacing = 32 mm"
equation "d200 = buttonHoleLength"
equation "d201 = buttonHoleWidth"
equation "d206 = buttonHoleLength"
equation "d207 = buttonHoleWidth"
equation "d208 = buttonHoleWidth"
equation "d209 = buttonHoleLength"
equation "ledOffset = 47 mm + wallThickness"
equation "ledWidth = 3 mm"
equation "d215 = ledWidth"
equation "d216 = ledHeight"
equation "buttonWall = 1 mm"
equation "buttonTopOffset = 5.5 mm"
equation "d225 = buttonHoleTopOffset"
equation "buttonHoleTopOffset = wallThickness - buttonWall + buttonTopOffset"
equation "d227 = buttonHoleTopOffset"
equation "buttonBottomOffset = 5.7 mm"
equation "buttonHoleBottomOffset = wallThickness - buttonWall + buttonBottomOffset"
equation "d230 = buttonHoleBottomOffset"
equation "d231 = buttonHoleBottomOffset"
equation "d237 = ledOffset"
equation "screenBevel = 1.5 mm"
equation "ledHeight = 3.6 mm"
equation "buttonHoleInset = 0.4 mm"
equation "d241 = buttonHoleInset"
equation "d242 = buttonHoleInset"
equation "d243 = buttonHoleInset"
equation "d244 = buttonHoleInset"
equation "d245 = buttonHoleInset"
equation "d246 = buttonHoleInset"
equation "d247 = buttonHoleInset"
equation "d248 = buttonHoleInset"
equation "d249 = buttonHoleInset"
equation "d250 = buttonHoleInset"
equation "d251 = buttonHoleInset"
equation "d252 = buttonHoleInset"
equation "screenDepth = 2.2 mm"
equation "d254 = topThickness"
equation "d256 = topThickness"
equation "d258 = -tabHeight"
equation "buttonInsetDepth = 2.8 mm"
equation "d261 = buttonInsetDepth"
equation "visibleScreenHeight = 16.5 mm"
equation "d265 = visibleScreenHeight"
equation "d266 = visibleScreenWidth"
equation "d268 = screenDepth"
equation "d271 = buttonInsetDepth"
equation "d274 = buttonInsetDepth"
equation "d277 = buttonInsetDepth"
equation "d290 = -tabHeight"
equation "d292 = -tabHeight"
equation "d294 = -tabHeight"
equation "d296 = -tabHeight"
equation "d298 = -tabHeight"
equation "d300 = mountID"
equation "d301 = mountOD"
equation "d302 = mountOD / 2"
equation "d303 = mountOD / 2"
equation "d304 = mountOD"
equation "d305 = mountID"
equation "d306 = mountOD / 2"
equation "d307 = mountOD / 2"
equation "topMountLength = topThickness - mountPlaneThickness"
equation "mountPlaneThickness = 2 mm"
equation "d310 = topMountLength"
equation "d312 = topMountLength"
equation "buttonHeight = 5.6 mm"
equation "buttonLipHeight = 2.3 mm"
equation "buttonLipThickness = 0.5 mm"
equation "d343 = mountID"
equation "d345 = mountID"
equation "d347 = mountID"
equation "d349 = mountID"
equation "buttonRightOffset = 8.3 mm"
equation "d354 = buttonRightOffset"
equation "d356 = screenLeftOffset"
equation "d358 = screenDepth"
equation "d435 = cornerRadius"
equation "d437 = cornerRadius"
equation "d439 = cornerRadius"
equation "d441 = cornerRadius"
named bodies: "Base", "Top", "Button"
